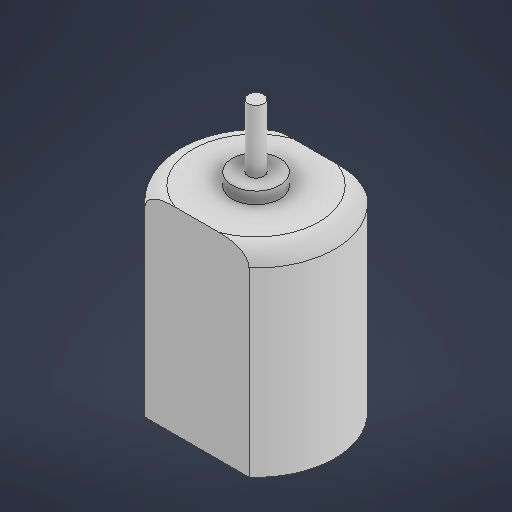
# Autodesk Inventor part: Pumpe
Saved by Autodesk Inventor 2026.2 (Build 302298000, 298)
## iProperties
Created: 2026-03-18
Part Number: Pumpe
Material: Generic
Document SubType Name: Modeling
Designer: Cobble
Density: 1 g/cm^3
Appearance: Default
Author: Cobble
Autodesk Inventor part; units mm, degrees
ref_plane "YZ Plane" through (0, 0, 0) normal (1, 0, 0) x (0, 1, 0)
ref_plane "XZ Plane" through (0, 0, 0) normal (0, 1, 0) x (-1, 0, 0)
ref_plane "XY Plane" through (0, 0, 0) normal (0, 0, 1) x (1, 0, 0)
sketch "Sketch1" plane through (0, 0, 0) normal (0, 0, 1) x (1, 0, 0)
  circle A0 centre (0, 0) radius 10
  line L0 (-10, -7.5) -> (-10, 7.5)
  line L1 (-10, 7.5) -> (10, 7.5)
  line L2 (10, 7.5) -> (10, -7.5)
  line L3 (10, -7.5) -> (-10, -7.5)
  line L4 (-10, -7.5) -> (10, 7.5) construction
  line L5 (-10, 7.5) -> (10, -7.5) construction
  circle A1 centre (0, 0) radius 3
  circle A2 centre (0, 0) radius 1
  point P0 (-6.6144, -7.5)
  point P1 (6.6144, -7.5)
  point P2 (6.6144, 7.5)
  point P3 (-6.6144, 7.5)
  dimension "d0" = 20
  dimension "d1" = 15
  dimension "d2" = 6
  dimension "d3" = 2
  constraints: 12 end point, 3 centre point, 3 coincident, 2 midpoint, 2 parallel, 1 perpendicular, 1 vertical
  measures "d0" diameter of A0
  measures "d1" distance of L0.start L0.end
  measures "d2" diameter of A1
  measures "d3" diameter of A2
extrude "Extrusion1" add sketch "Sketch1" along normal blind 1.5 contours A1
extrude "Extrusion2" add sketch "Sketch1" along normal blind 9.5 contours A2
extrude "Extrusion3" add sketch "Sketch1" against normal blind 25 contours A0 L3 L1 | A1 | A2
fillet "Fillet1" radius 2 2 edges at (-10, 0, 0) (10, 0, 0)
body "Solid1"
